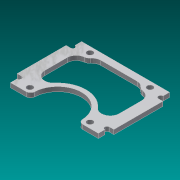
# Autodesk Inventor part: 足首_サブフレーム_1_1
Saved by Autodesk Inventor 2016 (Build 200138000, 138)
## iProperties
Created: 2016-04-30
Part Number: 足首_サブフレーム_1_1
Material: アルミニウム 2014-T4
Document SubType Name: Modeling
Designer: hiroaki
Density: 2.8 g/cm^3
Appearance: サテン
Mass: 3.0689 g
Surface Area: 17.0555 cm^2
Volume: 1.09604 cm^3
Author: hiroaki
Autodesk Inventor part; units mm, degrees
ref_plane "YZ Plane" through (0, 0, 0) normal (1, 0, 0) x (0, 1, 0)
ref_plane "XZ Plane" through (0, 0, 0) normal (0, 1, 0) x (-1, 0, 0)
ref_plane "XY Plane" through (0, 0, 0) normal (0, 0, 1) x (1, 0, 0)
sketch "スケッチ1" plane through (0, 0, 0) normal (0, 0, 1) x (1, 0, 0)
  circle A0 centre (0, 0) radius 10.5 construction
  circle A1 centre (-13.5, 1) radius 1.35
  line L0 (-13.5, 28) -> (13.5, 28) construction
  line L1 (13.5, 28) -> (13.5, 1) construction
  line L2 (13.5, 1) -> (-13.5, 1) construction
  line L3 (-13.5, 1) -> (-13.5, 28) construction
  circle A2 centre (-13.5, 28) radius 1.35
  circle A3 centre (13.5, 1) radius 1.35
  circle A4 centre (13.5, 28) radius 1.35
  line L4 (-19.75, 30.5) -> (-19.75, 27.6)
  line L5 (-19.75, 30.5) -> (19.75, 30.5)
  line L6 (19.75, 30.5) -> (19.75, 27.6)
  line L7 (-19.75, 1.4) -> (-19.75, -1.5)
  line L8 (-19.75, -1.5) -> (-10.6448, -1.5)
  line L9 (19.75, 1.4) -> (19.75, -1.5)
  line L10 (19.75, -1.5) -> (10.6448, -1.5)
  line L11 (-19.75, 25.5) -> (-21.75, 25.5)
  line L12 (-21.75, 25.5) -> (-21.75, 3.5)
  line L13 (-21.75, 3.5) -> (-19.75, 3.5)
  arc A5 (-19.75, 25.5) -> (-19.75, 27.6) centre (-19.75, 26.55) ccw
  arc A6 (-19.75, 1.4) -> (-19.75, 3.5) centre (-19.75, 2.45) ccw
  line L14 (19.75, 25.5) -> (21.75, 25.5)
  line L15 (21.75, 25.5) -> (21.75, 3.5)
  line L16 (21.75, 3.5) -> (19.75, 3.5)
  arc A7 (19.75, 27.6) -> (19.75, 25.5) centre (19.75, 26.55) ccw
  line L17 (0, 28) -> (0, 0) construction
  arc A8 (19.75, 3.5) -> (19.75, 1.4) centre (19.75, 2.45) ccw
  line L18 (-13.5, 14.5) -> (-21.75, 14.5) construction
  arc A9 (10.6448, -1.5) -> (-10.6448, -1.5) centre (0, 0) ccw
  point P0 (0, 30.5)
  dimension "d8" = 21
  dimension "d10" = 27
  dimension "d12" = 1
  dimension "d13" = 2.7
  dimension "d38" = 27
  dimension "d44" = 27
  dimension "d47" = 1.05
  dimension "d48" = 39.5
  dimension "d49" = 2
  dimension "d50" = 5
  dimension "d51" = 32
  dimension "d52" = 5
  dimension "d53" = 10.75
  constraints: 38 end point, 11 perpendicular, 10 centre point, 10 point on circle, 7 vertical alignment, 5 vertical, 4 horizontal, 4 midpoint, 4 tangent, 3 coincident, 3 equal radius, 3 symmetric about line, 2 parallel, 1 horizontal alignment, 7 other
  measures "d8" diameter of A0
  measures "d10" distance of L0.start L0.end
  measures "d12" distance from line of point (0, 0) L2
  measures "d13" diameter of A1
  measures "d38" distance of A1.centre A2.centre
  measures "d44" distance of A1.centre A3.centre
  measures "d47" radius of A5
  measures "d48" distance of L4.start L5.end
  measures "d49" distance between parallel lines of L12 L4
  measures "d50" distance between parallel lines of L8 L13
  measures "d51" distance between parallel lines of L8 L5
  measures "d52" distance between parallel lines of L5 L11
  measures "d53" radius of A9
extrude "押し出し1" add sketch "スケッチ1" along normal blind 2
sketch "スケッチ2" plane through (0, 0, 2) normal (0, 0, 1) x (1, 0, 0)
  circle A0 centre (13.5, 28) radius 1.35 projected
  circle A1 centre (-13.5, 28) radius 1.35 projected
  circle A2 centre (-13.5, 1) radius 1.35 projected
  line L0 (-19.75, 30.5) -> (-19.75, 27.6) projected
  arc A3 (10.6448, -1.5) -> (-10.6448, -1.5) centre (0, 0) ccw projected
  line L1 (19.75, 30.5) -> (-19.75, 30.5) projected
  line L2 (-10.542, 27.5) -> (10.542, 27.5)
  line L3 (-16.75, 25) -> (-16.75, 5)
  line L4 (16.75, 25) -> (16.75, 5)
  line L5 (-16.75, 5) -> (-11.7287, 5)
  line L6 (16.75, 5) -> (11.7287, 5)
  arc A4 (11.7287, 5) -> (-11.7287, 5) centre (0, 0) ccw
  line L7 (-16.75, 25) -> (-13.5, 25)
  arc A5 (-13.5, 25) -> (-10.542, 27.5) centre (-13.5, 28) ccw
  line L8 (16.75, 25) -> (13.5, 25)
  arc A6 (10.542, 27.5) -> (13.5, 25) centre (13.5, 28) ccw
  line L9 (0, 30.5) -> (0, 0) construction
  dimension "d56" = 2
  dimension "d57" = 4
  dimension "d58" = 3
  dimension "d59" = 3
  dimension "d60" = 3
  constraints: 16 end point, 6 point on circle, 4 horizontal, 3 centre point, 3 coincident, 3 vertical, 2 tangent, 1 equal radius, 1 horizontal alignment, 1 midpoint, 1 perpendicular, 1 other
  measures "d56" radial gap between concentric circles of A4 A3
  measures "d57" distance from line of A2.centre L5
  measures "d58" distance between parallel lines of L0 L3
  measures "d59" radius of A5
  measures "d60" distance between parallel lines of L1 L2
extrude "押し出し2" cut sketch "スケッチ2" against normal blind 10 contours L2 A6 L8 L4 L6 A4 L5 L3 L7 A5
fillet "フィレット1" radius 4 8 edges at (10.542, 27.5, 1) (16.75, 25, 1) (16.75, 5, 1) (11.7287, 5, 1) (-11.7287, 5, 1) (-16.75, 5, 1) (-16.75, 25, 1) (-10.542, 27.5, 1)
fillet "フィレット1" radius 2 2 edges at (-10.6448, -1.5, 1) (10.6448, -1.5, 1)
equation "\"d38\" = d10"
equation "\"d44\" = d10"
equation "\"d50\" = d30"
equation "\"d51\" = d18 + 2 * d30"
equation "\"d52\" = d50"
equation "\"d30\" = 5"
equation "\"d18\" = 22"
